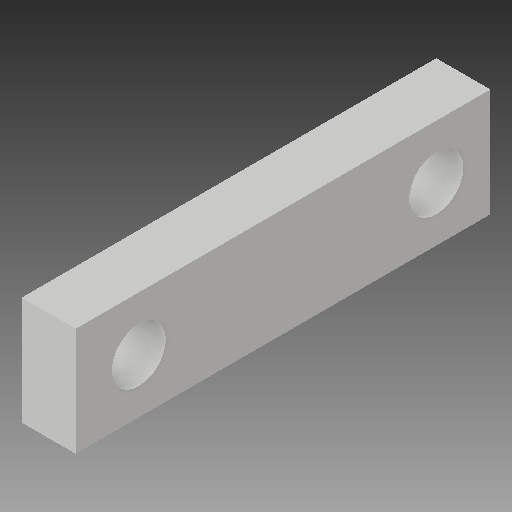
# Autodesk Inventor part: Bearing crossbar
Saved by Autodesk Inventor 2018 (Build 220112000, 112)
## iProperties
Created: 2018-06-26
Part Number: Bearing crossbar
Material: Generic
Document SubType Name: Modeling
Designer: Ajith Thomas
Density: 1 g/cm^3
Appearance: Default
Author: Ajith Thomas
Autodesk Inventor part; units mm, degrees
ref_plane "YZ Plane" through (0, 0, 0) normal (1, 0, 0) x (0, 1, 0)
ref_plane "XZ Plane" through (0, 0, 0) normal (0, 1, 0) x (-1, 0, 0)
ref_plane "XY Plane" through (0, 0, 0) normal (0, 0, 1) x (1, 0, 0)
sketch "Sketch1" plane through (0, 0, 0) normal (0, 0, 1) x (1, 0, 0)
  line L0 (1.5, 3) -> (4.5, 3) projected
  line L1 (4.5, 3) -> (4.5, -3) projected
  line L2 (4.5, -3) -> (1.5, -3) projected
  line L3 (1.5, -3) -> (1.5, 3) projected
  point P0 (0, 0)
extrude "Extrusion1" add sketch "Sketch1" along normal blind 8 and the other way blind 15
sketch "Sketch2" plane through (4.5, -3, 8) normal (1, 0, 0) x (0, 0, -1)
  circle A0 centre (3.5, 3) radius 1.5
  circle A1 centre (20, 3) radius 1.5
  line L0 (8, 7.2683) -> (8, -1.2683) construction
  point P0 (8, 3)
  dimension "d4" = 3
  dimension "d5" = 3
  dimension "d6" = 12
  dimension "d7" = 4.5
  constraints: 2 centre point
  measures "d4" diameter of A0
  measures "d5" diameter of A1
  measures "d6" distance from line of L0 A1.centre
  measures "d7" distance from line of L0 A0.centre
extrude "Extrusion2" cut sketch "Sketch2" against normal blind 8
body "Solid1"
